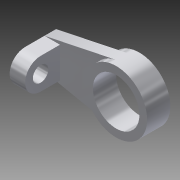
# Autodesk Inventor part: HW 7 Part 4
Saved by Autodesk Inventor 2015 (Build 190159000, 159)
## iProperties
Created: 2016-02-24
Part Number: HW 7 Part 4
Material: Aluminum 6061
Document SubType Name: Modeling
Designer: Melissa
Density: 2.7 g/cm^3
Appearance: Aluminum - Flat
Mass: 806.247 g
Surface Area: 513.658 cm^2
Volume: 298.61 cm^3
Author: Melissa
Autodesk Inventor part; units mm, degrees
ref_plane "YZ Plane" through (0, 0, 0) normal (1, 0, 0) x (0, 1, 0)
ref_plane "XZ Plane" through (0, 0, 0) normal (0, 1, 0) x (-1, 0, 0)
ref_plane "XY Plane" through (0, 0, 0) normal (0, 0, 1) x (1, 0, 0)
sketch "Sketch1" plane through (0, 0, 0) normal (0, 0, 1) x (1, 0, 0)
  circle A0 centre (0, 0) radius 38.1
  circle A1 centre (0, 0) radius 50.8
  line L0 (-127, 25.4) -> (-127, -25.4)
  line L1 (-127, 25.4) -> (-10.3741, 49.7294)
  line L2 (-127, -25.4) -> (-10.3741, -49.7294)
  dimension "d5" = 76.2
  dimension "d6" = 101.6
  dimension "d7" = 50.8
  dimension "d8" = 127
  dimension "d9" = 25.4
  constraints: 6 end point, 2 centre point, 2 coincident, 2 point on circle, 2 tangent, 1 vertical
  measures "d5" diameter of A0
  measures "d6" diameter of A1
  measures "d7" distance of L0.start L0.end
  measures "d8" distance from line of point (0, 0) L0
  measures "d9" vertical distance of point (0, 0) L0.start
extrude "Extrusion1" add sketch "Sketch1" along normal mid plane 19.05
extrude "Extrusion2" add sketch "Sketch1" along normal mid plane 38.1 contours A1
sketch "Sketch3" plane through (-127, -25.4, 9.525) normal (-1, 0, 0) x (0, 0, 1)
  line L0 (0, 50.8) -> (31.75, 50.8)
  line L1 (0, 0) -> (31.75, 0)
  arc A0 (31.75, 0) -> (31.75, 50.8) centre (31.75, 25.4) ccw
  line L2 (-19.05, 0) -> (-19.05, 50.8) projected
  circle A1 centre (31.75, 25.4) radius 12.7
  line L3 (0, 50.8) -> (0, 0)
  line L4 (0, 50.8) -> (-19.05, 50.8) projected
  point P0 (-9.525, 25.4)
  dimension "d14" = 25.4
  dimension "d15" = 50.8
  dimension "d16" = 25.4
  constraints: 6 end point, 2 centre point, 2 point on circle, 1 coincident, 1 horizontal, 1 parallel, 1 perpendicular, 1 tangent
  measures "d14" radius of A0
  measures "d15" distance from line of A0.centre L2
  measures "d16" diameter of A1
extrude "Extrusion3" add sketch "Sketch3" against normal blind 25.4
body "Solid1"
